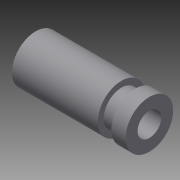
# Autodesk Inventor part: NozzleHolder
Saved by Autodesk Inventor 2014 SP1 (Build 180222100, 222)
## iProperties
Created: 2013-12-29
Part Number: NozzleHolder
Material: Polyethylene, High Density
Document SubType Name: Modeling
Designer: Jack
Density: 0.952 g/cm^3
Appearance: Smooth - Off-White
Author: Jack
Autodesk Inventor part; units mm, degrees
ref_plane "YZ Plane" through (0, 0, 0) normal (1, 0, 0) x (0, 1, 0)
ref_plane "XZ Plane" through (0, 0, 0) normal (0, 1, 0) x (-1, 0, 0)
ref_plane "XY Plane" through (0, 0, 0) normal (0, 0, 1) x (1, 0, 0)
sketch "Sketch1" plane through (0, 0, 0) normal (0, 1, 0) x (-1, 0, 0)
  line L0 (0, 4) -> (0, 8)
  line L1 (0, 8) -> (4.8, 8)
  line L2 (4.8, 8) -> (4.8, 6)
  line L3 (4.8, 6) -> (9.4, 6)
  line L4 (9.4, 6) -> (9.4, 8)
  line L5 (9.4, 8) -> (38.2679, 8)
  line L6 (0, 4) -> (7.5, 4)
  line L7 (7.5, 4) -> (7.5, 3.25)
  line L8 (40, 4) -> (36.8, 4)
  line L9 (36.8, 4) -> (36.8, 3.25)
  line L10 (40, 4) -> (40, 5)
  line L11 (38.2679, 8) -> (40, 5)
  line L12 (36.8, 3.25) -> (7.5, 3.25)
  line L13 (0, 0) -> (40, 0) construction
  dimension "d0" = 8
  dimension "d1" = 4.8
  dimension "d3" = 4.6
  dimension "d10" = 2
  dimension "d11" = 2
  dimension "d12" = 7.5
  dimension "d13" = 4
  dimension "d14" = 3.25
  dimension "d15" = 3.2
  dimension "d16" = 4
  dimension "d19" = 3.25
  dimension "d20" = 120
  dimension "d21" = 40
  dimension "d22" = 5
  dimension "d23" = 40
  constraints: 28 end point, 5 parallel, 4 perpendicular, 1 collinear, 1 horizontal, 1 vertical, 1 vertical alignment
  measures "d0" distance of L13.start L0.end
  measures "d1" distance of L0.end L1.end
  measures "d3" distance of L2.end L3.end
  measures "d10" distance of L3.end L4.end
  measures "d11" distance of L1.end L2.end
  measures "d12" distance of L0.start L6.end
  measures "d13" distance from line of L13.start L6
  measures "d14" vertical distance of L13.start L7.end
  measures "d15" distance of L8.start L8.end
  measures "d16" distance from line of L13.start L8
  measures "d19" vertical distance of L13.start L9.end
  measures "d20" angle of L5 L11
  measures "d21" distance between parallel lines of L0 L10
  measures "d22" vertical distance of L13.start L10.end
  measures "d23" distance of L13.start L13.end
revolve "Revolution1" add sketch "Sketch1" angle 360 about axis through (0, 0, 0) along (-1, 0, 0)
body "Solid1"
